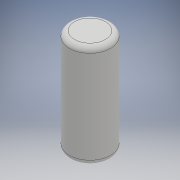
# Autodesk Inventor part: CP Pin d4
Saved by Autodesk Inventor 2017 (Build 210142000, 142)
## iProperties
Created: 2016-09-16
Part Number: CP Pin d4
Material: Generic
Document SubType Name: Modeling
Designer: Andreas Fröderberg
Density: 1 g/cm^3
Appearance: Default
Author: Andreas Fröderberg
Autodesk Inventor part; units mm, degrees
ref_plane "YZ Plane" through (0, 0, 0) normal (1, 0, 0) x (0, 1, 0)
ref_plane "XZ Plane" through (0, 0, 0) normal (0, 1, 0) x (-1, 0, 0)
ref_plane "XY Plane" through (0, 0, 0) normal (0, 0, 1) x (1, 0, 0)
sketch "Sketch1" plane through (0, 0, 0) normal (0, 0, 1) x (1, 0, 0)
  circle A0 centre (0, 0) radius 2
  dimension "d0" = 4
  constraints: 1 centre point, 1 coincident
  measures "d0" diameter of A0
extrude "Extrusion1" add sketch "Sketch1" along normal blind 10
fillet "Fillet1" radius 0.5 2 edges at (-2, 0, 10) (-2, 0, 0)
body "Solid1"
